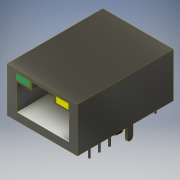
# Autodesk Inventor part: RJMG2012119A0NR_GBEConn
Saved by Autodesk Inventor 2016 (Build 200138000, 138)
## iProperties
Created: 2017-03-04
Part Number: RJMG2012119A0NR_GBEConn
Material: Generic
Document SubType Name: Modeling
Designer: jfixelle
Density: 1 g/cm^3
Appearance: Silver
Author: jfixelle
Autodesk Inventor part; units mm, degrees
ref_plane "YZ Plane" through (0, 0, 0) normal (1, 0, 0) x (0, 1, 0)
ref_plane "XZ Plane" through (0, 0, 0) normal (0, 1, 0) x (-1, 0, 0)
ref_plane "XY Plane" through (0, 0, 0) normal (0, 0, 1) x (1, 0, 0)
sketch "Sketch1" plane through (0, 0, 0) normal (0, 1, 0) x (-1, 0, 0)
  line L0 (8.89, 22.35) -> (-8.89, 22.35)
  line L1 (-8.89, 22.35) -> (-8.89, -1.78)
  line L2 (-8.89, -1.78) -> (8.89, -1.78)
  line L3 (8.89, -1.78) -> (8.89, 22.35)
  point P0 (0, 0)
  dimension "d0" = 24.13
  dimension "d1" = 22.35
  dimension "d2" = 17.78
  dimension "d3" = 8.89
  constraints: 8 end point, 2 parallel, 1 horizontal, 1 perpendicular
  measures "d0" distance of L2.end L0.start
  measures "d1" distance from line of point (0, 0) L0
  measures "d2" distance of L1.end L2.end
  measures "d3" distance from line of point (0, 0) L3
extrude "Extrusion1" add sketch "Sketch1" along normal blind 11.25
sketch "Sketch2" plane through (-8.89, 0, 22.35) normal (0, 0, 1) x (1, 0, 0)
  line L0 (2.4376, 1.9143) -> (15.6231, 1.9143)
  line L1 (15.6231, 1.9143) -> (15.6231, 8.5296)
  line L2 (15.6231, 8.5296) -> (2.4376, 8.5296)
  line L3 (2.4376, 8.5296) -> (2.4376, 1.9143)
  line L4 (6.2307, 8.5296) -> (11.6268, 8.5296)
  line L5 (11.6268, 8.5296) -> (11.6268, 10.4036)
  line L6 (11.6268, 10.4036) -> (6.2307, 10.4036)
  line L7 (6.2307, 10.4036) -> (6.2307, 8.5296)
  point P0 (8.89, 0)
  constraints: 16 end point, 4 parallel, 2 horizontal, 2 perpendicular, 1 point on line
extrude "Extrusion2" cut sketch "Sketch2" against normal blind 8
sketch "Sketch3" plane through (-8.89, 0, 22.35) normal (0, 0, 1) x (1, 0, 0)
  line L0 (12.4503, 9.0228) -> (15.6135, 9.0228)
  line L1 (15.6135, 9.0228) -> (15.6135, 10.4036)
  line L2 (15.6135, 10.4036) -> (12.4503, 10.4036)
  line L3 (12.4503, 10.4036) -> (12.4503, 9.0228)
  line L4 (5.8403, 9.0228) -> (2.4376, 9.0228)
  line L5 (2.4376, 9.0228) -> (2.4376, 10.4036)
  line L6 (2.4376, 10.4036) -> (5.8403, 10.4036)
  line L7 (5.8403, 10.4036) -> (5.8403, 9.0228)
  point P0 (8.89, 0)
  constraints: 16 end point, 4 parallel, 2 horizontal, 2 perpendicular, 2 point on line
extrude "Extrusion3" add sketch "Sketch3" along normal blind 0.1
sketch "Sketch4" plane through (8.89, 0, 22.35) normal (1, 0, 0) x (0, 0, -1)
  line L0 (12.46, 3.4608) -> (13.96, 3.4608)
  line L1 (13.96, 3.4608) -> (13.96, -3.3)
  line L2 (13.96, -3.3) -> (12.46, -3.3)
  line L3 (12.46, -3.3) -> (12.46, 3.4608)
  line L4 (0, 0) -> (0, 11.25) projected
  arc A0 (12.46, -2.55) -> (13.96, -2.55) centre (13.21, -2.55) ccw
  point P0 (22.35, 0)
  dimension "d10" = 1.5
  dimension "d11" = 12.46
  dimension "d12" = 3.3
  constraints: 8 end point, 3 tangent, 2 parallel, 2 point on circle, 2 point on line, 1 centre point, 1 horizontal, 1 perpendicular
  measures "d10" distance of L1.end L2.end
  measures "d11" distance between parallel lines of L4 L3
  measures "d12" distance from line of L2 point (22.35, 0)
extrude "Extrusion4" add sketch "Sketch4" against normal blind 0.5 contours L0 L1 A0 L3
mirror "Mirror1" about plane through (0, 0, 0) normal (1, 0, 0) of "Extrusion4"
sketch "Sketch5" plane through (0, 0, 0) normal (0, -1, 0) x (1, 0, 0)
  circle A0 centre (-4.825, 9.14) radius 1.675
  circle A1 centre (4.825, 9.14) radius 1.675
  line L0 (-8.89, 22.35) -> (8.89, 22.35) projected
  point P0 (0, 0)
  dimension "d15" = 9.65
  dimension "d16" = 4.825
  dimension "d17" = 13.21
  dimension "d18" = 13.21
  dimension "d19" = 3.35
  dimension "d20" = 3.35
  constraints: 2 centre point
  measures "d15" distance of A1.centre A0.centre
  measures "d16" horizontal distance of point (0, 0) A1.centre
  measures "d17" distance from line of L0 A1.centre
  measures "d18" distance from line of L0 A0.centre
  measures "d19" diameter of A1
  measures "d20" diameter of A0
extrude "Extrusion5" add sketch "Sketch5" along normal blind 3.3
chamfer "Chamfer1" distance 0.5 angle 45 2 edges at (-6.5, -3.3, 9.14) (3.15, -3.3, 9.14)
sketch "Sketch6" plane through (0, 0, 0) normal (0, -1, 0) x (1, 0, 0)
  line L0 (-9.0913, 0) -> (4.8455, 0) construction
  line L1 (4.957, 2.54) -> (-8.5338, 2.54) construction
  circle A0 centre (-2.03, 0) radius 0.25
  circle A1 centre (-1.015, 2.54) radius 0.25
  line L2 (-11.1213, 0) -> (2.8155, 0) construction
  circle A2 centre (-3.045, 2.54) radius 0.25
  line L3 (-13.1513, 0) -> (0.7855, 0) construction
  circle A3 centre (-5.075, 2.54) radius 0.25
  circle A4 centre (1.015, 2.54) radius 0.25
  circle A5 centre (3.045, 2.54) radius 0.25
  circle A6 centre (5.075, 2.54) radius 0.25
  circle A7 centre (-4.06, 0) radius 0.25
  circle A8 centre (-6.09, 0) radius 0.25
  line L4 (0, 0) -> (0, 4.0434) construction
  circle A9 centre (2.03, 0) radius 0.25
  circle A10 centre (4.06, 0) radius 0.25
  circle A11 centre (6.09, 0) radius 0.25
  point P0 (-4.06, 0)
  point P1 (-6.09, 0)
  dimension "d26" = 0.5
  dimension "d27" = 0.5
  dimension "d28" = 2.54
  dimension "d29" = 1.015
  dimension "d30" = 1.015
  dimension "d33" = 2.03
  dimension "d40" = 2.03
  dimension "d47" = 2.03
  constraints: 12 centre point, 10 end point, 5 horizontal, 4 point on line, 3 symmetric about line, 1 vertical, 25 other
  measures "d26" diameter of A1
  measures "d27" diameter of A0
  measures "d28" distance between parallel lines of L0 L1
  measures "d29" horizontal distance of L4.start A1.centre
  measures "d30" horizontal distance of A0.centre A1.centre
  measures "d33" distance of L0.start L2.start
  measures "d40" distance of A1.centre A4.centre
  measures "d47" distance of A0.centre A7.centre
extrude "Extrusion6" add sketch "Sketch6" along normal blind 3.18
sketch "Sketch7" plane through (0, 0, 0) normal (0, -1, 0) x (1, 0, 0)
  line L0 (7.52, 20.8101) -> (7.52, 18.5144) construction
  line L1 (-7.52, 21.4502) -> (-7.52, 19.3214) construction
  line L2 (-8.1276, 18.03) -> (7.9812, 18.03) construction
  line L3 (-8.0282, 15.49) -> (8.0806, 15.49) construction
  circle A0 centre (-7.52, 18.03) radius 0.25
  circle A1 centre (-7.52, 15.49) radius 0.25
  circle A2 centre (7.52, 18.03) radius 0.25
  circle A3 centre (7.52, 15.49) radius 0.25
  circle A4 centre (7.52, 12.95) radius 0.25
  point P0 (0, 0)
  dimension "d54" = 7.52
  dimension "d55" = 15.04
  dimension "d56" = 0.5
  dimension "d57" = 0.5
  dimension "d58" = 0.5
  dimension "d59" = 0.5
  dimension "d60" = 0.5
  dimension "d61" = 18.03
  dimension "d62" = 2.54
  dimension "d63" = 2.54
  constraints: 9 point on line, 8 end point, 5 centre point, 2 horizontal, 2 vertical
  measures "d54" distance from line of point (0, 0) L1
  measures "d55" distance between parallel lines of L0 L1
  measures "d56" diameter of A2
  measures "d57" diameter of A3
  measures "d58" diameter of A4
  measures "d59" diameter of A0
  measures "d60" diameter of A1
  measures "d61" distance from line of point (0, 0) L2
  measures "d62" distance from line of A4.centre L3
  measures "d63" distance of A2.centre A3.centre
extrude "Extrusion7" add sketch "Sketch7" along normal blind 3.18
body "Solid1"
